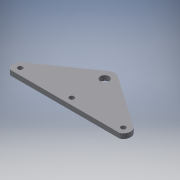
# Autodesk Inventor part: Corpo_Suporte_3_Cabos_Modelo2
Saved by Autodesk Inventor 2018 (Build 220112000, 112)
## iProperties
Created: 2021-08-02
Part Number: Corpo_Suporte_3_Cabos_Modelo2
Material: Generic
Document SubType Name: Modeling
Designer: L08619
Density: 1 g/cm^3
Appearance: Default
Author: L08619
Autodesk Inventor part; units mm, degrees
ref_plane "YZ Plane" through (0, 0, 0) normal (1, 0, 0) x (0, 1, 0)
ref_plane "XZ Plane" through (0, 0, 0) normal (0, 1, 0) x (-1, 0, 0)
ref_plane "XY Plane" through (0, 0, 0) normal (0, 0, 1) x (1, 0, 0)
sketch "Sketch1" plane through (0, 0, 0) normal (0, 0, 1) x (1, 0, 0)
  circle A0 centre (0, 0) radius 20
  circle A1 centre (-235, -150) radius 11
  arc A2 (-254.009, -122.9246) -> (-248.9435, -180) centre (-235, -150) ccw
  line L0 (-254.009, -122.9246) -> (-20, 40)
  line L1 (-20, 40) -> (-10, 46.2314) construction
  spline S0 degree 2 poles (-20, 40) (-10, 46.2314) (0, 46.2314) knots 1 1 1 1.5 1.5 1.5
  line L2 (0, 107.1559) -> (0, -270.9336) construction
  line L3 (-10, 46.2314) -> (0, 46.2314) construction
  circle A3 centre (235, -150) radius 11
  arc A4 (248.9435, -180) -> (254.009, -122.9246) centre (235, -150) ccw
  line L4 (254.009, -122.9246) -> (20, 40)
  line L5 (20, 40) -> (10, 46.2314) construction
  spline S1 degree 2 poles (20, 40) (10, 46.2314) (0, 46.2314) knots 1 1 1 1.5 1.5 1.5
  line L6 (10, 46.2314) -> (0, 46.2314) construction
  circle A5 centre (0, -150) radius 11
  line L7 (248.9435, -180) -> (-248.9435, -180)
  dimension "d0" = 40
  dimension "d3" = 22
  dimension "d9" = 40
  dimension "d12" = 120
  dimension "d18" = 22
  dimension "d19" = 150
  constraints: 8 end point, 6 centre point, 6 symmetric about line, 4 point on circle, 3 coincident, 2 horizontal alignment, 2 point on line, 1 horizontal, 1 vertical, 8 other
  measures "d0" diameter of A0
  measures "d3" diameter of A1
  measures "d9" vertical distance of L0.end point (0, 0)
  measures "d18" diameter of A5
  measures "d19" distance of point (0, 0) A5.centre
extrude "Extrusion2" add sketch "Sketch1" along normal mid plane 22.22
equation "\"d18\" = d3"
body "Solid2"
